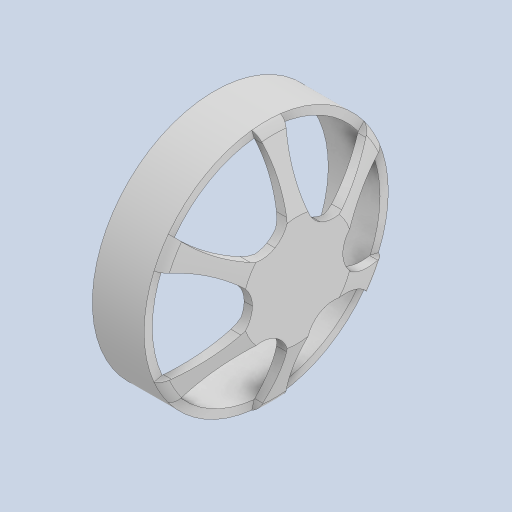
# Autodesk Inventor part: mot_4006_shell
Saved by Autodesk Inventor 2023 (Build 270158000, 158)
## iProperties
Created: 2022-10-31
Part Number: mot_4006_shell
Material: Generic
Document SubType Name: Modeling
Designer: Shuang Peng
Density: 1 g/cm^3
Appearance: Default
Author: Shuang Peng
Autodesk Inventor part; units mm, degrees
ref_plane "YZ Plane" through (0, 0, 0) normal (1, 0, 0) x (0, 1, 0)
ref_plane "XZ Plane" through (0, 0, 0) normal (0, 1, 0) x (-1, 0, 0)
ref_plane "XY Plane" through (0, 0, 0) normal (0, 0, 1) x (1, 0, 0)
sketch "Sketch1" plane through (0, 0, 0) normal (0, 1, 0) x (-1, 0, 0)
  line L0 (0, 0) -> (171.313, 0) construction
  line L1 (171.313, 0) -> (171.313, -170.0373) construction
  line L2 (171.313, -170.0373) -> (0, -170.0373) construction
  line L3 (0, -170.0373) -> (0, 0) construction
  line L4 (0, 22.175) -> (0, -22.175)
  line L5 (0, 22.175) -> (-9.4, 22.175)
  line L6 (0, -22.175) -> (-9.4, -22.175)
  line L7 (-9.4, -22.175) -> (-9.4, 22.175)
  line L8 (-9.4, 0) -> (-15.1, 0)
  line L9 (-15.1, 0) -> (-15.1, -10)
  line L10 (-9.4, -22.175) -> (-9.4, -20.775)
  line L11 (-9.4, -20.775) -> (-10.8, -20.775)
  line L12 (-15.1, -10) -> (-10.8, -20.775)
  arc A0 (-10.8, -20.775) -> (-9.4, -22.175) centre (-8.4703, -19.8453) ccw
  line L13 (-9.4, 0) -> (0, 0)
  dimension "d9" = 44.35
  dimension "d16" = 9.4
  dimension "d19" = 5.7
  dimension "d20" = 10
  dimension "d21" = 1.4
  dimension "d22" = 1.4
  constraints: 20 end point, 3 horizontal, 2 midpoint, 2 perpendicular, 2 point on circle, 2 vertical, 1 centre point, 1 point on line, 1 tangent, 2 other
  measures "d9" distance of L4.start L4.end
  measures "d16" distance of L4.start L5.end
  measures "d19" distance of L8.start L8.end
  measures "d20" distance of L8.end L9.end
  measures "d21" distance of L6.end L10.end
  measures "d22" distance of L10.end L11.end
revolve "Revolution1" add sketch "Sketch1" angle 360 about axis through (9.4, 0, 0) along (-1, 0, 0) contours L4 L6 L7 L13 | L7 L11 L12 L9 L8 | A0 L11 L7
sketch "Sketch2" plane through (15.1, 0, 0) normal (1, 0, 0) x (0, 0, -1)
  line L0 (-136.091, 48.5097) -> (38.0121, 48.5097) construction
  line L1 (38.0121, 48.5097) -> (38.0121, -124.2969) construction
  line L2 (38.0121, -124.2969) -> (-136.091, -124.2969) construction
  line L3 (-136.091, -124.2969) -> (-136.091, 48.5097) construction
  circle A0 centre (0, 0) radius 20.5
  line L4 (0, 0) -> (-20.5, 0)
  line L5 (0, 0) -> (-18.7277, -8.3381)
  line L6 (0, 0) -> (20.5, 0) construction
  line L7 (-20.5, 0) -> (-10, 0)
  circle A1 centre (0, 0) radius 10 projected
  line L8 (-10, 0) -> (-10, -3.8)
  arc A2 (-18.7277, -8.3381) -> (-10, -3.8) centre (-24.2562, 12.9559) ccw
  line L9 (-10, 0) -> (-8.2, 0)
  arc A3 (-10, -3.8) -> (-8.2, 0) centre (-13.1998, 0.042) ccw
  arc A4 (-10, 3.8) -> (-18.7277, 8.3381) centre (-24.2562, -12.9559) ccw
  arc A5 (-8.2, 0) -> (-10, 3.8) centre (-13.1998, -0.042) ccw
  line L10 (-18.7277, -8.3381) -> (-20.3761, -8.7491)
  circle A6 centre (0, 0) radius 22.175 projected
  line L11 (-18.7277, 8.3381) -> (-20.3761, 8.7491)
  point P0 (-20.3761, 8.7491)
  dimension "d37" = 41
  dimension "d38" = 20.5
  dimension "d39" = 156
  dimension "d40" = 10.5
  dimension "d41" = 3.8
  dimension "d42" = 22
  dimension "d43" = 1.8
  dimension "d44" = 5
  dimension "d53" = 170
  constraints: 16 end point, 8 point on circle, 5 symmetric about line, 4 centre point, 2 horizontal, 2 horizontal alignment, 2 point on line, 1 coincident, 1 equal length, 1 vertical, 8 other
  measures "d38" distance of L4.start L5.end
  measures "d39" angle of L5 L6
  measures "d40" distance of L4.end L7.end
  measures "d41" distance of L7.end L8.end
  measures "d42" radius of A2
  measures "d43" distance of L7.end L9.end
  measures "d44" radius of A3
  measures "d53" angle of L5 L10
extrude "Extrusion1" cut sketch "Sketch2" against normal blind 5.7 contours A4 A5 A1 L4 A0 | A0 L10 A6 L11 | A0 L4 L8 A2 L5 | L5 A2 | A1 A5 L4 | L4 A3 A1 | A1 A3 L8 picked at (-21.3987, -2.4397)
pattern_circular "Circular Pattern1" count 6 over 360 about axis through (4.7, 0, 0) along (-1, 0, 0) of "Extrusion1"
sketch "Sketch3" plane through (0, 0, 0) normal (0, 0, 1) x (1, 0, 0)
  line L0 (15.1, 0) -> (9.4, 0) projected
  line L1 (15.1, 0) -> (13.6, 0)
  line L2 (13.6, 0) -> (13.6, -9)
  line L3 (14.8216, -10.5603) -> (9.4, -10.5603) projected
  line L4 (0, 22.175) -> (0, -22.175) projected
  line L5 (0, -22.175) -> (0, -20.675)
  line L6 (0, -20.675) -> (9.4, -20.675)
  line L7 (9.4, -13.2716) -> (9.4, -22.0207) projected
  line L8 (9.4, -20.675) -> (13.6, -9)
  line L9 (13.6, 0) -> (0, 0)
  line L10 (0, 0) -> (0, -20.675)
  dimension "d61" = 1.5
  dimension "d62" = 9
  dimension "d63" = 1.5
  constraints: 14 end point, 4 perpendicular, 3 point on line
  measures "d61" distance of L0.start L1.end
  measures "d62" distance of L1.end L2.end
  measures "d63" distance of L4.end L5.end
revolve "Revolution2" cut sketch "Sketch3" angle 360 about axis through (13.6, 0, 0) along (-1, 0, 0)
body "Solid1"
